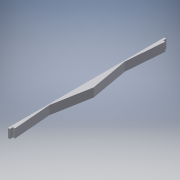
# Autodesk Inventor part: long_insert_inv
Saved by Autodesk Inventor 2017 (Build 210142000, 142)
## iProperties
Created: 2018-01-14
Part Number: long_insert_inv
Material: Generic
Document SubType Name: Modeling
Designer: Mitch
Density: 1 g/cm^3
Appearance: White
Author: Mitch
Autodesk Inventor part; units mm, degrees
ref_plane "YZ Plane" through (0, 0, 0) normal (1, 0, 0) x (0, 1, 0)
ref_plane "XZ Plane" through (0, 0, 0) normal (0, 1, 0) x (-1, 0, 0)
ref_plane "XY Plane" through (0, 0, 0) normal (0, 0, 1) x (1, 0, 0)
sketch "Sketch1" plane through (0, 0, 0) normal (0, 1, 0) x (-1, 0, 0)
  line L0 (0, 0) -> (0, -125.2474)
  line L1 (0, -125.2474) -> (-3.4036, -125.2474)
  line L2 (0, 0) -> (-3.4036, 0)
  line L3 (-3.4036, 0) -> (-0.889, -31.2039)
  line L4 (-0.889, -31.2039) -> (-6.5786, -62.4078)
  line L5 (-6.5786, -62.4078) -> (-0.889, -94.0308)
  line L6 (-0.889, -94.0308) -> (-3.4036, -125.2474)
  dimension "d0" = 125.2474
  dimension "d1" = 3.4036
  dimension "d2" = 3.4036
  dimension "d3" = 31.2039
  dimension "d4" = 62.4078
  dimension "d5" = 31.2166
  dimension "d15" = 6.5786
  dimension "d16" = 0.889
  dimension "d17" = 0.889
  constraints: 14 end point, 2 horizontal, 1 vertical
  measures "d0" distance of L0.start L0.end
  measures "d1" distance of L0.end L1.end
  measures "d2" distance of L0.start L2.end
  measures "d3" vertical distance of L3.end L2.end
  measures "d4" vertical distance of L4.end L2.end
  measures "d5" vertical distance of L5.end L1.end
  measures "d15" distance from line of L0 L4.end
  measures "d16" distance from line of L0 L3.end
  measures "d17" distance from line of L0 L5.end
extrude "Extrusion1" add sketch "Sketch1" along normal blind 7.3025
sketch "Sketch2" plane through (0, 0, 0) normal (0, 0, 1) x (1, 0, 0)
  line L0 (3.4036, 0) -> (0, 0) projected
  line L1 (0, 7.3025) -> (1.651, 7.3025)
  line L2 (1.651, 7.3025) -> (1.651, 0)
  line L3 (1.651, 0) -> (0, 0)
  line L4 (0, 0) -> (0, 7.3025)
  dimension "d8" = 1.651
  constraints: 8 end point, 2 parallel, 1 horizontal, 1 perpendicular, 1 point on line
  measures "d8" distance of L2.end L3.end
sketch "Sketch3" plane through (3.4036, 0, -125.2474) normal (0, 0, -1) x (-1, 0, 0)
  line L0 (3.4036, 0) -> (3.4036, 7.3025) projected
  line L1 (0, 0) -> (3.4036, 0) projected
  line L2 (3.4036, 7.3025) -> (1.7526, 7.3025)
  line L3 (1.7526, 7.3025) -> (1.7526, 0)
  line L4 (1.7526, 0) -> (3.4036, 0)
  line L5 (3.4036, 0) -> (3.4036, 7.3025)
  dimension "d9" = 1.651
  constraints: 8 end point, 2 parallel, 1 horizontal, 1 perpendicular, 1 point on line
  measures "d9" distance of L4.end L3.end
extrude "Extrusion2" add sketch "Sketch3" along normal blind 2.5654
extrude "Extrusion3" add sketch "Sketch2" along normal blind 2.5654
body "Solid1"
